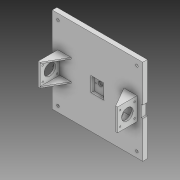
# Autodesk Inventor part: Topper
Saved by Autodesk Inventor 2020 (Build 240168000, 168)
## iProperties
Created: 2020-10-19
Part Number: Topper
Material: Generic
Document SubType Name: Modeling
Designer: DDeGo
Density: 1 g/cm^3
Appearance: Default
Author: DDeGo
Autodesk Inventor part; units mm, degrees
ref_plane "YZ Plane" through (0, 0, 0) normal (1, 0, 0) x (0, 1, 0)
ref_plane "XZ Plane" through (0, 0, 0) normal (0, 1, 0) x (-1, 0, 0)
ref_plane "XY Plane" through (0, 0, 0) normal (0, 0, 1) x (1, 0, 0)
sketch "Sketch1" plane through (0, 0, 0) normal (0, 0, 1) x (1, 0, 0)
  line L0 (-97.5, -92.5) -> (97.5, -92.5)
  line L1 (97.5, -92.5) -> (97.5, 92.5)
  line L2 (97.5, 92.5) -> (-97.5, 92.5)
  line L3 (-97.5, 92.5) -> (-97.5, -92.5)
  line L4 (-97.5, -92.5) -> (97.5, 92.5) construction
  line L5 (97.5, -92.5) -> (-97.5, 92.5) construction
  line L6 (85, -80) -> (-85, -80) construction
  line L7 (-85, -80) -> (-85, 80) construction
  line L8 (-85, 80) -> (85, 80) construction
  line L9 (85, 80) -> (85, -80) construction
  line L10 (85, -80) -> (-85, 80) construction
  line L11 (-85, -80) -> (85, 80) construction
  line L12 (-95.15, 89.5529) -> (-74.85, 89.5529)
  line L13 (-74.85, 89.5529) -> (-74.85, 70.4471)
  line L14 (-74.85, 70.4471) -> (-95.15, 70.4471)
  line L15 (-95.15, 70.4471) -> (-95.15, 89.5529)
  line L16 (-95.15, 89.5529) -> (-74.85, 70.4471) construction
  line L17 (-74.85, 89.5529) -> (-95.15, 70.4471) construction
  line L18 (95.15, 89.5529) -> (74.85, 89.5529)
  line L19 (74.85, 89.5529) -> (74.85, 70.4471)
  line L20 (74.85, 70.4471) -> (95.15, 70.4471)
  line L21 (95.15, 70.4471) -> (95.15, 89.5529)
  line L22 (95.15, 89.5529) -> (74.85, 70.4471) construction
  line L23 (74.85, 89.5529) -> (95.15, 70.4471) construction
  line L24 (95.15, -89.5529) -> (74.85, -89.5529)
  line L25 (74.85, -89.5529) -> (74.85, -70.4471)
  line L26 (74.85, -70.4471) -> (95.15, -70.4471)
  line L27 (95.15, -70.4471) -> (95.15, -89.5529)
  line L28 (95.15, -89.5529) -> (74.85, -70.4471) construction
  line L29 (74.85, -89.5529) -> (95.15, -70.4471) construction
  line L30 (-95.15, -89.5529) -> (-74.85, -89.5529)
  line L31 (-74.85, -89.5529) -> (-74.85, -70.4471)
  line L32 (-74.85, -70.4471) -> (-95.15, -70.4471)
  line L33 (-95.15, -70.4471) -> (-95.15, -89.5529)
  line L34 (-95.15, -89.5529) -> (-74.85, -70.4471) construction
  line L35 (-74.85, -89.5529) -> (-95.15, -70.4471) construction
  point P0 (0, 0)
  dimension "d0" = 195
  dimension "d1" = 20.3
  dimension "d2" = 170
  dimension "d23" = 185
  dimension "d24" = 160
  constraints: 72 end point, 12 midpoint, 12 parallel, 6 horizontal, 6 perpendicular, 5 point on line, 3 equal length
  measures "d0" distance of L1.end L2.end
  measures "d1" distance of L12.start L12.end
  measures "d2" distance of L7.end L8.end
  measures "d23" distance of L0.end L1.end
  measures "d24" distance of L6.end L7.end
extrude "Extrusion1" add sketch "Sketch1" along normal blind 5
sketch "Sketch2" plane through (0, 0, 5) normal (0, 0, 1) x (1, 0, 0)
  line L0 (97.5, 92.5) -> (-97.5, 92.5) projected
  line L1 (97.5, -92.5) -> (-97.5, -92.5)
  line L2 (-97.5, -92.5) -> (-97.5, 92.5)
  line L3 (-97.5, 92.5) -> (97.5, 92.5)
  line L4 (97.5, 92.5) -> (97.5, -92.5)
  line L5 (97.5, -92.5) -> (-97.5, 92.5) construction
  line L6 (-97.5, -92.5) -> (97.5, 92.5) construction
  line L7 (-74.85, 70.4471) -> (-95.15, 70.4471) construction
  line L8 (-74.85, 89.5529) -> (-74.85, 70.4471) construction
  line L9 (-95.15, 70.4471) -> (-74.85, 89.5529) construction
  line L10 (74.85, 89.5529) -> (95.15, 89.5529) projected
  line L11 (95.15, 70.4471) -> (74.85, 70.4471) construction
  line L12 (74.85, 89.5529) -> (95.15, 70.4471) construction
  line L13 (74.85, -70.4471) -> (95.15, -70.4471) construction
  line L14 (74.85, -89.5529) -> (74.85, -70.4471) construction
  line L15 (95.15, -70.4471) -> (74.85, -89.5529) construction
  line L16 (-74.85, -89.5529) -> (-95.15, -89.5529) construction
  line L17 (-95.15, -89.5529) -> (-95.15, -70.4471) projected
  line L18 (-74.85, -89.5529) -> (-95.15, -70.4471) construction
  circle A0 centre (-85, 80) radius 2.75
  circle A1 centre (85, 80) radius 2.75
  circle A2 centre (85, -80) radius 2.75
  circle A3 centre (-85, -80) radius 2.75
  point P0 (0, 0)
  dimension "d7" = 5.5
  constraints: 16 end point, 4 centre point, 4 midpoint, 3 equal radius, 2 parallel, 1 horizontal, 1 perpendicular, 8 other
  measures "d7" diameter of A0
extrude "Extrusion2" add sketch "Sketch2" along normal blind 5
sketch "Sketch3" plane through (0, 0, 10) normal (0, 0, 1) x (1, 0, 0)
  line L0 (0, 0) -> (-96, 0) construction
  line L1 (0, 0) -> (96, 0) construction
  line L2 (-97.5, -12.5) -> (-94.5, -12.5)
  line L3 (-94.5, -12.5) -> (-94.5, 12.5)
  line L4 (-94.5, 12.5) -> (-97.5, 12.5)
  line L5 (-97.5, 12.5) -> (-97.5, -12.5)
  line L6 (-97.5, -12.5) -> (-94.5, 12.5) construction
  line L7 (-94.5, -12.5) -> (-97.5, 12.5) construction
  line L8 (94.5, -12.5) -> (97.5, -12.5)
  line L9 (97.5, -12.5) -> (97.5, 12.5)
  line L10 (97.5, 12.5) -> (94.5, 12.5)
  line L11 (94.5, 12.5) -> (94.5, -12.5)
  line L12 (94.5, -12.5) -> (97.5, 12.5) construction
  line L13 (97.5, -12.5) -> (94.5, 12.5) construction
  circle A0 centre (-85, 80) radius 2.75 projected
  line L14 (-85, 80) -> (-96, 0) construction
  circle A1 centre (85, 80) radius 2.75 projected
  line L15 (-97.5, 92.5) -> (-97.5, -92.5) projected
  dimension "d8" = 3
  dimension "d9" = 25
  constraints: 30 end point, 4 horizontal, 4 midpoint, 4 parallel, 3 equal length, 2 perpendicular, 1 point on line
  measures "d8" distance of L3.end L4.end
  measures "d9" distance of L2.end L3.end
extrude "Extrusion3" cut sketch "Sketch3" against normal through all contours L5 L4 L3 L2 | L11 L10 L9 L8
sketch "Sketch4" plane through (0, 0, 10) normal (0, 0, 1) x (1, 0, 0)
  line L0 (0, 0) -> (83.5, 0) construction
  line L1 (0, 0) -> (-83.5, 0) construction
  line L2 (-85.5, -21.15) -> (-81.5, -21.15)
  line L3 (-81.5, -21.15) -> (-81.5, 21.15)
  line L4 (-81.5, 21.15) -> (-85.5, 21.15)
  line L5 (-85.5, 21.15) -> (-85.5, -21.15)
  line L6 (-85.5, -21.15) -> (-81.5, 21.15) construction
  line L7 (-81.5, -21.15) -> (-85.5, 21.15) construction
  line L8 (81.5, -21.15) -> (85.5, -21.15)
  line L9 (85.5, -21.15) -> (85.5, 21.15)
  line L10 (85.5, 21.15) -> (81.5, 21.15)
  line L11 (81.5, 21.15) -> (81.5, -21.15)
  line L12 (81.5, -21.15) -> (85.5, 21.15) construction
  line L13 (85.5, -21.15) -> (81.5, 21.15) construction
  line L14 (-94.5, 12.5) -> (-94.5, -12.5) projected
  dimension "d13" = 42.3
  dimension "d14" = 4
  dimension "d22" = 13
  constraints: 28 end point, 4 horizontal, 4 midpoint, 4 parallel, 2 collinear, 2 perpendicular, 1 point on line
  measures "d13" distance of L2.end L3.end
  measures "d14" distance of L3.end L4.end
  measures "d22" distance between parallel lines of L14 L3
extrude "Extrusion4" add sketch "Sketch4" along normal blind 42.3
sketch "Sketch5" plane through (-85.5, -21.15, 10) normal (-1, 0, 0) x (0, 0, 1)
  line L0 (0, 0) -> (0, 42.3) projected
  line L1 (0, 0) -> (42.3, 0) projected
  line L2 (42.3, 42.3) -> (42.3, 0) projected
  line L3 (0, 42.3) -> (42.3, 42.3) projected
  line L4 (36.65, 5.65) -> (5.65, 5.65) construction
  line L5 (5.65, 5.65) -> (5.65, 36.65) construction
  line L6 (5.65, 36.65) -> (36.65, 36.65) construction
  line L7 (36.65, 36.65) -> (36.65, 5.65) construction
  line L8 (36.65, 36.65) -> (5.65, 5.65) construction
  circle A0 centre (36.65, 36.65) radius 1.75
  circle A1 centre (36.65, 5.65) radius 1.75
  circle A2 centre (21.15, 21.15) radius 12.5
  circle A3 centre (5.65, 5.65) radius 1.75
  circle A4 centre (5.65, 36.65) radius 1.75
  point P0 (-10, 21.15)
  dimension "d17" = 31
  dimension "d18" = 3.5
  dimension "d19" = 25
  constraints: 10 end point, 5 centre point, 4 coincident, 3 equal radius, 1 midpoint, 3 other
  measures "d17" distance of L6.end L4.start
  measures "d18" diameter of A1
  measures "d19" diameter of A2
extrude "Extrusion5" cut sketch "Sketch5" against normal through all contours A0 | A1 | A2 | A3 | A4
sketch "Sketch8" plane through (-85.5, -21.15, 10) normal (0, -1, 0) x (1, 0, 0)
  line L0 (4, 0) -> (0, 0) projected
  line L1 (4, 0) -> (4, 42.3) construction
  line L2 (0, 42.3) -> (4, 42.3) projected
  line L3 (0, 0) -> (0, 42.3) projected
  line L4 (171, 0) -> (167, 0) projected
  line L5 (171, 0) -> (171, 42.3) projected
  line L6 (167, 42.3) -> (171, 42.3) projected
  line L7 (167, 0) -> (167, 42.3) construction
  line L8 (4, 42.3) -> (28.4219, 0)
  line L9 (-12, 0) -> (183, 0) construction
  line L10 (4, 0) -> (28.4219, 0)
  line L11 (171, 42.3) -> (167, 42.3) projected
  line L12 (167, 42.3) -> (142.5781, 0)
  line L13 (142.5781, 0) -> (167, 0)
  point P0 (85.5, -10)
  dimension "d30" = 60
  dimension "d31" = 60
  constraints: 8 end point, 2 collinear, 2 point on line
  measures "d30" angle of L9 L8
  measures "d31" angle of L9 L12
extrude "Extrusion8" add sketch "Sketch8" along normal blind 3
mirror "Mirror1" about plane through (0, 0, 0) normal (0, 1, 0) of "Extrusion8"
ref_plane "Work Plane2" through (0, 0, 3.5) normal (0, 0, -1) x (-1, 0, 0)
sketch "Sketch6" plane through (0, 0, 10) normal (0, 0, 1) x (1, 0, 0)
  circle A0 centre (0, 0) radius 5
  dimension "d25" = 10
  constraints: 1 centre point, 1 coincident
  measures "d25" diameter of A0
extrude "Extrusion6" cut sketch "Sketch6" against normal through all
sketch "Sketch7" plane through (0, 0, 10) normal (0, 0, 1) x (1, 0, 0)
  circle A0 centre (0, 0) radius 5 projected
  line L0 (-14, 12) -> (14, 12)
  line L1 (14, 12) -> (14, -20)
  line L2 (14, -20) -> (-14, -20)
  line L3 (-14, -20) -> (-14, 12)
  dimension "d34" = 28
  dimension "d35" = 14
  dimension "d36" = 12
  dimension "d37" = 20
  constraints: 8 end point, 2 parallel, 1 horizontal, 1 perpendicular
  measures "d34" distance between parallel lines of L1 L3
  measures "d35" distance from line of L3 point (0, 0)
  measures "d36" distance from line of A0.centre L0
  measures "d37" distance from line of L2 A0.centre
extrude "Extrusion7" cut sketch "Sketch7" against normal up to surface (6.5 mm away)
sketch "Sketch9" plane through (-14, 12, 3.5) normal (0, 0, 1) x (1, 0, 0)
  circle A0 centre (24.25, -3) radius 1.2
  line L0 (24.25, -15.5) -> (24.25, -3) construction
  circle A1 centre (24.25, -15.5) radius 1.2
  line L1 (24.25, -3) -> (3.75, -3) construction
  circle A2 centre (3.75, -3) radius 1.2
  line L2 (3.75, -15.5) -> (24.25, -15.5) construction
  line L3 (3.75, -15.5) -> (24.25, -3) construction
  line L4 (3.75, -3) -> (3.75, -15.5) construction
  line L5 (24.25, -15.5) -> (3.75, -3) construction
  circle A3 centre (3.75, -15.5) radius 1.2
  line L6 (0, 0) -> (28, 0) projected
  line L7 (14, -9.25) -> (14, 0) construction
  line L8 (28, 0) -> (0, 0) projected
  point P0 (14, -12)
  dimension "d39" = 2.4
  dimension "d40" = 12.5
  dimension "d41" = 20.5
  dimension "d42" = 3
  constraints: 14 end point, 4 centre point, 4 coincident, 3 equal radius, 3 midpoint, 2 parallel, 1 horizontal, 1 perpendicular, 1 vertical
  measures "d39" diameter of A3
  measures "d40" distance of L1.end L2.start
  measures "d41" distance of L2.start L0.start
  measures "d42" distance between parallel lines of L6 L1
extrude "Extrusion9" cut sketch "Sketch9" against normal through all
ref_plane "Work Plane1" through (0, 0, 0) normal (0, 1, 0) x (-1, 0, 0)
equation "\"d35\" = 0.5 * d34"
body "Solid1"
